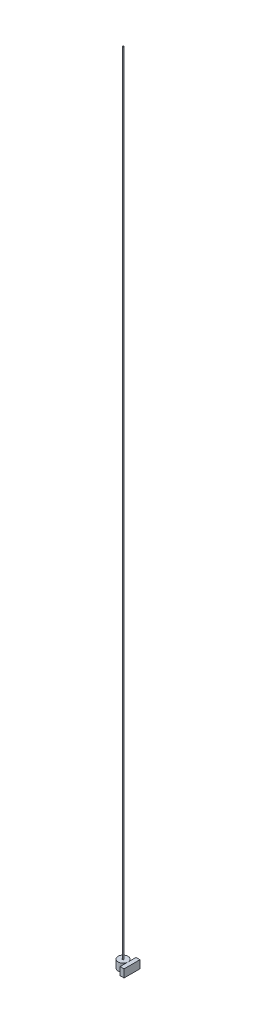
# Autodesk Inventor part: Laser
Saved by Autodesk Inventor 2026.2 (Build 302298000, 298)
## iProperties
Created: 2025-12-18
Part Number: Laser
Material: Generic
Document SubType Name: Modeling
Designer: Thoma
Density: 1 g/cm^3
Appearance: Default
Mass: 2.21776 g
Surface Area: 13.5699 cm^2
Volume: 2.21776 cm^3
Author: Thoma
Autodesk Inventor part; units mm, degrees
ref_plane "YZ Plane" through (0, 0, 0) normal (1, 0, 0) x (0, 1, 0)
ref_plane "XZ Plane" through (0, 0, 0) normal (0, 1, 0) x (-1, 0, 0)
ref_plane "XY Plane" through (0, 0, 0) normal (0, 0, 1) x (1, 0, 0)
sketch "Sketch1" plane through (0, 0, 0) normal (0, 1, 0) x (-1, 0, 0)
  circle A0 centre (11.25, 0) radius 6.25
  line L0 (5, 10) -> (0, 10)
  line L1 (0, 10) -> (0, -10)
  line L2 (0, -10) -> (5, -10)
  line L3 (5, -10) -> (5, 10)
  point P0 (0, 0)
  point P1 (2.5, -10)
  point P2 (2.5, 10)
  point P3 (5, 0)
  point P4 (5, 0)
  dimension "d0" = 10
  dimension "d1" = 10
  dimension "d2" = 0
  dimension "d3" = 12.5
  dimension "d4" = 5
  constraints: 8 end point, 3 midpoint, 2 parallel, 1 centre point, 1 horizontal, 1 perpendicular, 1 tangent
  measures "d0" vertical distance of point (2.5, -10) point (0, 0)
  measures "d1" vertical distance of point (2.5, 10) point (0, 0)
  measures "d2" vertical distance of point (5, 0) A0.centre
  measures "d3" diameter of A0
  measures "d4" distance between parallel lines of L3 L1
extrude "Extrusion1" add sketch "Sketch1" along normal blind 10
sketch "Sketch2" plane through (-11.25, 10, 0) normal (0, 1, 0) x (1, 0, 0)
  circle A0 centre (0, 0) radius 1
  point P0 (11.25, 0)
  constraints: 1 centre point
extrude "Extrusion2" cut sketch "Sketch2" against normal blind 3
sketch "Sketch3" plane through (-11.25, 7, 0) normal (0, 1, 0) x (1, 0, 0)
  circle A0 centre (0, 0) radius 0.75
  point P0 (11.25, 0)
  dimension "d9" = 1.5
  constraints: 1 centre point
  measures "d9" diameter of A0
extrude "Extrusion3" add sketch "Sketch3" along normal blind 1000
body "Solid1"
